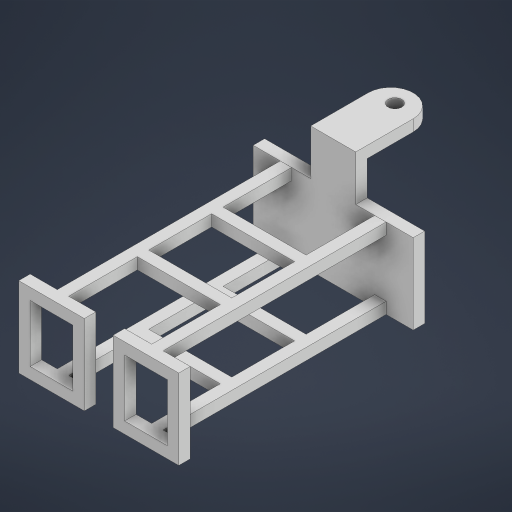
# Autodesk Inventor part: MHead
Saved by Autodesk Inventor 2024 (Build 280153000, 153)
## iProperties
Created: 2023-06-14
Part Number: MHead
Material: Generic
Document SubType Name: Modeling
Designer: vilas
Density: 1 g/cm^3
Appearance: Default
Author: vilas
Autodesk Inventor part; units mm, degrees
ref_plane "YZ Plane" through (0, 0, 0) normal (1, 0, 0) x (0, 1, 0)
sketch "Sketch1" plane through (0, 0, 0) normal (0, 0, 1) x (1, 0, 0)
  line L0 (-18.15, 12.5) -> (18.15, 12.5) construction
  line L1 (18.15, 12.5) -> (18.15, -12.5) construction
  line L2 (18.15, -12.5) -> (-18.15, -12.5) construction
  line L3 (-18.15, -12.5) -> (-18.15, 12.5) construction
  line L4 (-18.15, 12.5) -> (18.15, -12.5) construction
  line L5 (18.15, 12.5) -> (-18.15, -12.5) construction
  line L6 (-18.15, 12.5) -> (-23.15, 12.5)
  line L7 (-23.15, 12.5) -> (-23.15, 17.5)
  line L8 (-23.15, 17.5) -> (-18.15, 17.5)
  line L9 (-18.15, 17.5) -> (-18.15, 12.5)
  line L10 (18.15, 12.5) -> (23.15, 12.5)
  line L11 (23.15, 12.5) -> (23.15, 17.5)
  line L12 (23.15, 17.5) -> (18.15, 17.5)
  line L13 (18.15, 17.5) -> (18.15, 12.5)
  line L14 (18.15, -12.5) -> (23.15, -12.5)
  line L15 (23.15, -12.5) -> (23.15, -17.5)
  line L16 (23.15, -17.5) -> (18.15, -17.5)
  line L17 (18.15, -17.5) -> (18.15, -12.5)
  line L18 (-18.15, -12.5) -> (-23.15, -12.5)
  line L19 (-23.15, -12.5) -> (-23.15, -17.5)
  line L20 (-23.15, -17.5) -> (-18.15, -17.5)
  line L21 (-18.15, -17.5) -> (-18.15, -12.5)
  point P0 (0, 0)
  dimension "d0" = 36.3
  dimension "d1" = 25
  dimension "d2" = 5
  dimension "d3" = 5
  dimension "d4" = 5
  dimension "d5" = 5
  dimension "d6" = 5
  dimension "d7" = 5
  dimension "d8" = 5
  dimension "d9" = 5
  constraints: 44 end point, 10 parallel, 5 horizontal, 5 perpendicular, 2 midpoint
  measures "d0" distance of L1.end L2.end
  measures "d1" distance of L0.end L1.end
  measures "d2" distance of L7.end L8.end
  measures "d3" distance of L6.end L7.end
  measures "d4" distance of L12.end L11.end
  measures "d5" distance of L11.end L10.end
  measures "d6" distance of L15.end L16.end
  measures "d7" distance of L14.end L15.end
  measures "d8" distance of L20.end L19.end
  measures "d9" distance of L19.end L18.end
extrude "Extrusion1" add sketch "Sketch1" along normal mid plane 97.524
ref_plane "Work Plane1" through (0, 0, 48.762) normal (0, 0, 1) x (1, 0, 0)
sketch "Sketch2" plane through (0, 0, 48.762) normal (0, 0, 1) x (1, 0, 0)
  line L0 (0, 0) -> (-20.65, 0) construction
  line L1 (0, 0) -> (20.65, 0) construction
  line L2 (-35, 17.5) -> (-6.3, 17.5)
  line L3 (-6.3, 17.5) -> (-6.3, -17.5)
  line L4 (-6.3, -17.5) -> (-35, -17.5)
  line L5 (-35, -17.5) -> (-35, 17.5)
  line L6 (-35, 17.5) -> (-6.3, -17.5) construction
  line L7 (-6.3, 17.5) -> (-35, -17.5) construction
  line L8 (6.3, 17.5) -> (35, 17.5)
  line L9 (35, 17.5) -> (35, -17.5)
  line L10 (35, -17.5) -> (6.3, -17.5)
  line L11 (6.3, -17.5) -> (6.3, 17.5)
  line L12 (6.3, 17.5) -> (35, -17.5) construction
  line L13 (35, 17.5) -> (6.3, -17.5) construction
  line L14 (-11.3, 12.5) -> (-30, 12.5)
  line L15 (-30, 12.5) -> (-30, -12.5)
  line L16 (-30, -12.5) -> (-11.3, -12.5)
  line L17 (-11.3, -12.5) -> (-11.3, 12.5)
  line L18 (30, 12.5) -> (11.3, 12.5)
  line L19 (11.3, 12.5) -> (11.3, -12.5)
  line L20 (11.3, -12.5) -> (30, -12.5)
  line L21 (30, -12.5) -> (30, 12.5)
  dimension "d13" = 20.65
  dimension "d14" = 20.65
  dimension "d15" = 28.7
  dimension "d16" = 35
  dimension "d17" = 28.7
  dimension "d18" = 35
  dimension "d19" = 5
  dimension "d20" = 5
  constraints: 44 end point, 8 parallel, 4 horizontal, 4 midpoint, 4 perpendicular, 6 other
  measures "d13" distance of L0.start L0.end
  measures "d14" distance of L0.start L1.end
  measures "d15" distance of L3.end L4.end
  measures "d16" distance of L2.end L3.end
  measures "d17" distance of L9.end L10.end
  measures "d18" distance of L8.end L9.end
  measures "d19" distance between parallel lines of L2 L14
  measures "d20" distance between parallel lines of L8 L18
extrude "Extrusion2" add sketch "Sketch2" along normal blind 5
ref_plane "Work Plane2" through (0, 0, -48.771) normal (0, 0, 1) x (1, 0, 0)
sketch "Sketch4" plane through (0, 0, 0) normal (1, 0, 0) x (0, 1, 0)
  line L0 (12.5, -48.762) -> (12.5, 48.762) projected
  line L1 (12.5, 18.754) -> (17.5, 18.754)
  line L2 (17.5, 18.754) -> (17.5, 13.754)
  line L3 (17.5, 13.754) -> (12.5, 13.754)
  line L4 (12.5, 13.754) -> (12.5, 18.754)
  line L5 (-12.5, 48.762) -> (12.5, 48.762) projected
  line L6 (12.5, -13.754) -> (17.5, -13.754)
  line L7 (17.5, -13.754) -> (17.5, -18.754)
  line L8 (17.5, -18.754) -> (12.5, -18.754)
  line L9 (12.5, -18.754) -> (12.5, -13.754)
  line L10 (17.5, -48.762) -> (12.5, -48.762) projected
  line L11 (-12.5, 48.762) -> (-12.5, -48.762) projected
  line L12 (-12.5, 18.754) -> (-17.5, 18.754)
  line L13 (-17.5, 18.754) -> (-17.5, 13.754)
  line L14 (-17.5, 13.754) -> (-12.5, 13.754)
  line L15 (-12.5, 13.754) -> (-12.5, 18.754)
  line L16 (-12.5, -18.754) -> (-17.5, -18.754)
  line L17 (-17.5, -18.754) -> (-17.5, -13.754)
  line L18 (-17.5, -13.754) -> (-12.5, -13.754)
  line L19 (-12.5, -13.754) -> (-12.5, -18.754)
  line L20 (-12.5, -48.762) -> (-17.5, -48.762) projected
  point P0 (0, 0)
  point P1 (-17.5, 48.762)
  point P2 (17.5, 48.762)
  point P3 (-12.5, 13.754)
  point P4 (12.5, 13.754)
  point P5 (-12.5, -13.754)
  dimension "d30" = 5
  dimension "d31" = 5
  dimension "d32" = 30.008
  dimension "d33" = 5
  dimension "d34" = 5
  dimension "d35" = 30.008
  dimension "d36" = 5
  dimension "d37" = 5
  dimension "d38" = 5
  dimension "d39" = 5
  dimension "d40" = 30.008
  dimension "d41" = 30.008
  constraints: 32 end point, 8 parallel, 4 horizontal, 4 perpendicular, 4 point on line
  measures "d30" distance of L2.end L3.end
  measures "d31" distance of L1.end L2.end
  measures "d32" distance between parallel lines of L1 L5
  measures "d33" distance of L7.end L8.end
  measures "d34" distance of L6.end L7.end
  measures "d35" distance between parallel lines of L8 L10
  measures "d36" distance of L14.end L13.end
  measures "d37" distance of L13.end L12.end
  measures "d38" distance of L17.end L18.end
  measures "d39" distance of L16.end L17.end
  measures "d40" distance between parallel lines of L16 L20
  measures "d41" distance between parallel lines of L12 L5
extrude "Extrusion4" add sketch "Sketch4" along normal mid plane 36.3
sketch "Sketch7" plane through (0, 0, -48.771) normal (0, 0, 1) x (1, 0, 0)
  line L0 (0, 0) -> (0, 37.394) construction
  line L1 (0, 37.394) -> (9.85, 37.394) construction
  line L2 (9.85, 37.394) -> (-9.85, 37.394)
  line L3 (35, 17.5) -> (23.15, 17.5) projected
  line L4 (-35, -17.5) -> (-6.3, -17.5) projected
  line L5 (35, 17.5) -> (-35, 17.5)
  line L6 (-35, 17.5) -> (-35, -17.5)
  line L7 (-35, -17.5) -> (35, -17.5)
  line L8 (35, -17.5) -> (35, 17.5)
  line L9 (9.85, 37.394) -> (9.85, 17.5)
  line L10 (-9.85, 37.394) -> (-9.85, 17.5)
  dimension "d63" = 37.394
  dimension "d64" = 9.85
  constraints: 18 end point, 4 perpendicular, 2 horizontal, 2 parallel, 2 point on line, 1 vertical
  measures "d63" distance of L0.start L0.end
  measures "d64" distance of L0.end L1.end
extrude "Extrusion7" add sketch "Sketch7" against normal blind 5
sketch "Sketch8" plane through (0, 0, -53.771) normal (0, 0, -1) x (-1, 0, 0)
  line L0 (9.85, 17.5) -> (9.85, 37.394) projected
  line L1 (-9.85, 37.394) -> (9.85, 37.394)
  line L2 (9.85, 37.394) -> (9.85, 32.394)
  line L3 (9.85, 32.394) -> (-9.85, 32.394)
  line L4 (-9.85, 32.394) -> (-9.85, 37.394)
  point P0 (0, 0)
  dimension "d76" = 5
  constraints: 8 end point, 2 parallel, 1 horizontal, 1 perpendicular, 1 point on line
  measures "d76" distance of L1.end L2.end
extrude "Extrusion8" add sketch "Sketch8" along normal blind 30
fillet "Fillet2" radius 9.85 2 edges at (9.85, 34.894, -83.771) (-9.85, 34.894, -83.771)
sketch "Sketch10" plane through (-9.85, 32.394, -53.771) normal (0, -1, 0) x (1, 0, 0)
  circle A0 centre (9.85, -22) radius 3
  line L0 (44.85, 0) -> (-25.15, 0) projected
  point P0 (9.85, 53.771)
  dimension "d77" = 6
  dimension "d78" = 22
  constraints: 1 centre point
  measures "d77" diameter of A0
  measures "d78" distance from line of A0.centre L0
extrude "Extrusion10" cut sketch "Sketch10" against normal through all
body "Solid1"
